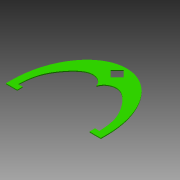
# Autodesk Inventor part: Patron
Saved by Autodesk Inventor 2015 SP1 (Build 190203100, 203)
## iProperties
Created: 2015-05-01
Part Number: Patron
Material: Générique
Document SubType Name: Modeling
Designer: Cyril
Density: 1 g/cm^3
Appearance: Default(1)
Author: Cyril
Autodesk Inventor part; units mm, degrees
ref_plane "YZ Plane" through (0, 0, 0) normal (1, 0, 0) x (0, 1, 0)
ref_plane "XZ Plane" through (0, 0, 0) normal (0, 1, 0) x (-1, 0, 0)
ref_plane "XY Plane" through (0, 0, 0) normal (0, 0, 1) x (1, 0, 0)
sketch "Sketch1" plane through (0, 0, 0) normal (0, 0, 1) x (1, 0, 0)
  arc A0 (105, 0) -> (-105, 0) centre (0, 0) ccw construction
  spline S0 degree 4 poles (-90, 0) (-89.8538, 2.5777) (-89.5214, 7.7436) (-88.895, 15.5264) (-87.5092, 26.0481) (-85.1483, 36.8225) (-81.2834, 47.9668) (-75.3893, 59.5396) (-67.7797, 71.1244) (-59.0389, 82.0507) (-49.6428, 91.5021) (-39.9949, 98.5099) (-30.4634, 101.9112) (-21.48, 101.6824) (-13.5876, 99.0404) (-7.4233, 95.0146) (-3.4101, 90.3959) (-1.5003, 86.7313) (-0.4634, 84.2499) (0, 83) knots 0 0 0 0 0 0.0625 0.125 0.1875 0.25 0.3125 0.375 0.4375 0.5 0.5625 0.625 0.6875 0.75 0.8125 0.875 0.9375 1 1 1 1 1
  line L0 (-14.1421, 129.1421) -> (0, 143.2843)
  line L1 (0, 143.2843) -> (14.1421, 129.1421)
  line L2 (14.1421, 129.1421) -> (0, 115)
  line L3 (0, 115) -> (-14.1421, 129.1421)
  line L4 (-80, -12) -> (-80, 0)
  line L5 (-80, 0) -> (-90, 0)
  ellipse E0 centre (0, 0) end of major axis (0, -150) minor radius 105 (105, 0) -> (-105, 0) ccw
  circle A1 centre (0, 45) radius 35 construction
  line L6 (-80, -12) -> (-105, -12)
  line L7 (-105, -12) -> (-105, 0)
  line L8 (-105, 0) -> (105, 0) construction
  line L9 (0, 0) -> (0, 150) construction
  spline S1 degree 4 poles (90, 0) (89.8538, 2.5777) (89.5214, 7.7436) (88.895, 15.5264) (87.5092, 26.0481) (85.1483, 36.8225) (81.2834, 47.9668) (75.3893, 59.5396) (67.7797, 71.1244) (59.0389, 82.0507) (49.6428, 91.5021) (39.9949, 98.5099) (30.4634, 101.9112) (21.48, 101.6824) (13.5876, 99.0404) (7.4233, 95.0146) (3.4101, 90.3959) (1.5003, 86.7313) (0.4634, 84.2499) (0, 83) knots 0 0 0 0 0 0.0625 0.125 0.1875 0.25 0.3125 0.375 0.4375 0.5 0.5625 0.625 0.6875 0.75 0.8125 0.875 0.9375 1 1 1 1 1
  line L10 (80, -12) -> (80, 0)
  line L11 (80, 0) -> (90, 0)
  line L12 (80, -12) -> (105, -12)
  line L13 (105, -12) -> (105, 0)
  point P0 (-80, 50)
  point P1 (-35, 100)
  point P2 (-8, 95)
  point P3 (80, 50)
  point P4 (35, 100)
  point P5 (8, 95)
  dimension "d0" = 105
  dimension "d1" = 20
  dimension "d2" = 20
  dimension "d7" = 12
  dimension "d8" = 10
  dimension "d20" = 70
  dimension "d30" = 50
  dimension "d31" = 100
  dimension "d32" = 95
  dimension "d33" = 83
  dimension "d34" = 45
  dimension "d35" = 150
  dimension "d36" = 115
  dimension "d37" = 8
  dimension "d38" = 35
  dimension "d39" = 80
  dimension "d40" = 90
  constraints: 28 end point, 7 symmetric about line, 4 point on line, 4 vertical, 2 centre point, 2 coincident, 2 collinear, 2 parallel, 2 perpendicular, 2 point on circle, 1 horizontal, 1 midpoint, 15 other
  measures "d0" radius of A0
  measures "d1" distance of L0.start L0.end
  measures "d2" distance of L2.end L0.start
  measures "d7" distance of L4.start L4.end
  measures "d8" distance of L4.end L5.end
  measures "d20" diameter of A1
  measures "d30" distance from line of L8 point (-80, 50)
  measures "d31" distance from line of L8 point (-35, 100)
  measures "d32" distance from line of L8 point (-8, 95)
  measures "d33" distance from line of L8 point (0, 83)
  measures "d34" distance from line of L8 A1.centre
  measures "d35" distance from line of L8 L9.end
  measures "d36" distance from line of L8 L2.end
  measures "d37" distance from line of L9 point (-8, 95)
  measures "d38" distance from line of L9 point (-35, 100)
  measures "d39" distance from line of L9 point (-80, 50)
  measures "d40" distance from line of L9 L5.end
extrude "Extrusion1" add sketch "Sketch1" along normal blind 2
equation "\"d2\" = d1"
body "Solid1"
